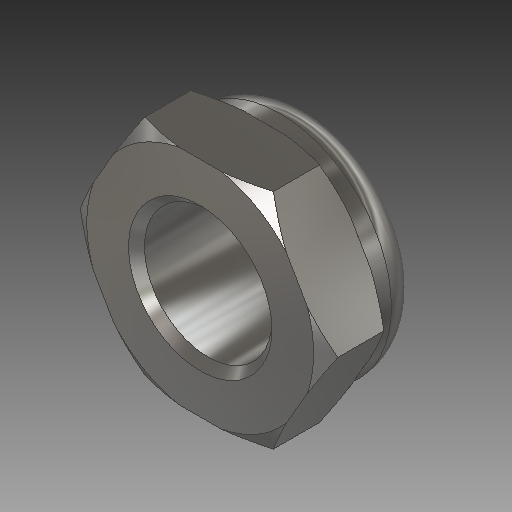
# Autodesk Inventor part: paris_nut
Saved by Autodesk Inventor 2019.3 (Build 233278000, 278)
## iProperties
Created: 2017-04-02
Part Number: paris_nut
Material: Типовые
Document SubType Name: Modeling
Designer: Nikita
Density: 1 g/cm^3
Appearance: Сталь — полированная
Mass: 0.742434 g
Surface Area: 6.80647 cm^2
Volume: 0.742434 cm^3
Author: Nikita
Autodesk Inventor part; units mm, degrees
ref_plane "YZ Plane" through (0, 0, 0) normal (1, 0, 0) x (0, 1, 0)
ref_plane "XZ Plane" through (0, 0, 0) normal (0, 1, 0) x (-1, 0, 0)
ref_plane "XY Plane" through (0, 0, 0) normal (0, 0, 1) x (1, 0, 0)
sketch "Эскиз1" plane through (0, 0, 0) normal (0, 0, 1) x (1, 0, 0)
  circle A0 centre (0, 0) radius 4
  line L0 (8.0829, 0) -> (4.0415, -7)
  line L1 (4.0415, -7) -> (-4.0415, -7)
  line L2 (-4.0415, -7) -> (-8.0829, 0)
  line L3 (-8.0829, 0) -> (-4.0415, 7)
  line L4 (-4.0415, 7) -> (4.0415, 7)
  line L5 (4.0415, 7) -> (8.0829, 0)
  dimension "d0" = 8
  dimension "d1" = 14
  constraints: 12 end point, 2 coincident, 1 centre point, 1 horizontal, 13 other
  measures "d0" diameter of A0
  measures "d1" distance between parallel lines of L1 L4
extrude "Выдавливание1" add sketch "Эскиз1" along normal blind 4
sketch "Эскиз2" plane through (0, 0, 0) normal (0, 1, 0) x (-1, 0, 0)
  line L0 (0, 0) -> (0, 12.9838)
  line L1 (-4.0415, 0) -> (-8.0829, 0) construction
  line L2 (-8.0829, 0) -> (-8.0829, 4) construction
  line L3 (-8.0829, 4) -> (-4.0415, 4) construction
  line L4 (-3.7273, -1.9581) -> (-10.5829, 2)
  line L5 (-10.5829, 2) -> (-3.7273, 5.9581)
  line L6 (-3.7273, 5.9581) -> (-11.5829, 5.9581)
  line L7 (-11.5829, 5.9581) -> (-11.5829, -1.9581)
  line L8 (-11.5829, -1.9581) -> (-3.7273, -1.9581)
  line L9 (-8.0829, 2) -> (-29.2681, 2) construction
  point P0 (-11.5829, 2)
  dimension "d4" = 60
  dimension "d5" = 1
  dimension "d6" = 3.5
  constraints: 14 end point, 2 horizontal, 2 midpoint, 2 perpendicular, 2 point on line, 1 vertical, 1 other
  measures "d4" angle of L5 L4
  measures "d5" distance from line of L7 L4.end
  measures "d6" distance between parallel lines of L2 L7
revolve "Вращение1" cut sketch "Эскиз2" angle 360 about axis through (0, 0, 0) along (0, 0, 1)
sketch "Эскиз3" plane through (0, 0, 0) normal (0, 0, -1) x (-1, 0, 0)
  line L0 (5.4146, -4.6216) -> (6.7097, -2.3784) construction
  circle A0 centre (0, 0) radius 7
  circle A1 centre (0, 0) radius 4 projected
  constraints: 1 centre point, 1 coincident, 1 tangent
extrude "Выдавливание2" add sketch "Эскиз3" along normal blind 3
fillet "Сопряжение1" radius 2 1 edges at (7, 0, -3)
sketch "Эскиз4" plane through (0, 0, -3) normal (0, 0, -1) x (-1, 0, 0)
  circle A0 centre (0, 0) radius 4 projected
  circle A1 centre (0, 0) radius 4.65
  dimension "d14" = 9.3
  constraints: 1 centre point, 1 coincident
  measures "d14" diameter of A1
extrude "Выдавливание3" cut sketch "Эскиз4" against normal blind 0.2
fillet "Сопряжение2" radius 0.2 1 edges at (4.65, 0, -3)
chamfer "Фаска2" distance 0.5 angle 45 1 edges at (-4, 0, 4)
